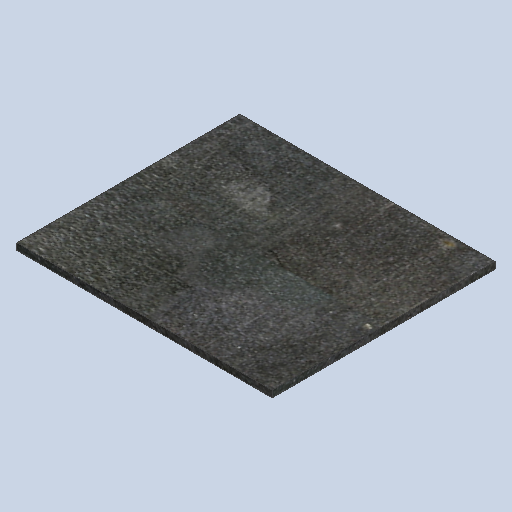
# Autodesk Inventor part: Flu-Expansion-RS3
Saved by Autodesk Inventor 2024.3 (Build 283343000, 343)
## iProperties
Created: 2025-06-18
Part Number: Flu-Expansion-RS3
Material: Steel
Document SubType Name: Modeling
Designer: ajclo
Density: 7.85 g/cm^3
Appearance: Plate
Mass: 269.775 g
Surface Area: 241.981 cm^2
Volume: 34.3662 cm^3
Author: ajclo
Autodesk Inventor part; units mm, degrees
ref_plane "YZ Plane" through (0, 0, 0) normal (1, 0, 0) x (0, 1, 0)
ref_plane "XZ Plane" through (0, 0, 0) normal (0, 1, 0) x (-1, 0, 0)
ref_plane "XY Plane" through (0, 0, 0) normal (0, 0, 1) x (1, 0, 0)
sketch "Sketch1" plane through (0, 0, 0) normal (0, 1, 0) x (-1, 0, 0)
  line L0 (57.277, 50) -> (-57.277, 50)
  line L1 (-57.277, 50) -> (-57.277, -50)
  line L2 (-57.277, -50) -> (57.277, -50)
  line L3 (57.277, -50) -> (57.277, 50)
  line L4 (57.277, 50) -> (-57.277, -50) construction
  line L5 (-57.277, 50) -> (57.277, -50) construction
  point P0 (0, 0)
  dimension "d0" = 100
  dimension "d1" = 114.554
  constraints: 12 end point, 2 midpoint, 2 parallel, 1 horizontal, 1 perpendicular
  measures "d0" distance of L2.end L0.start
  measures "d1" distance of L1.end L2.end
extrude "Extrusion1" add sketch "Sketch1" along normal blind 3
body "Solid1"
